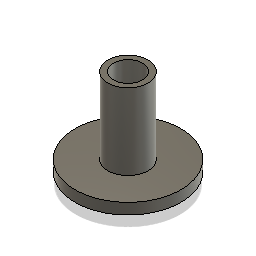
Rotor v1 (Autodesk Fusion 360 design; units mm, degrees)
Autodesk Fusion 360 part; units mm, degrees
note: some values were not read from the file. Set by a fixed rule: which sketch regions a step uses.
sketch "Esboço1" plane through (0, 0, 0) normal (0, 1, 0) x (1, 0, 0)
  circle A0 centre (0, 0) radius 14.5
  circle A1 centre (0, 0) radius 5.5
  circle A2 centre (0, 0) radius 4
  dimension "d1" = 29
  dimension "d2" = 11
  dimension "d3" = 8
  constraint coincident A0.centre A1.centre
  constraint concentric A0 A1
  measures "d1" diameter of A0
  measures "d2" diameter of A1
  measures "d3" diameter of A2
extrude "Extrusão1" add sketch "Esboço1" along normal blind 3 contours A0 makes body 1
extrude "Extrusão2" add sketch "Esboço1" against normal blind 3 separate body contours A1 makes body 2
extrude "Extrusão3" add sketch "Esboço1" along normal blind 23.8 contours A1 bodies 1 2
sketch "Esboço3" plane through (0, 0, 0) normal (0, 0, 1) x (1, 0, 0)
  line L0 (0, 0) -> (0, -7.7454)
  circle A0 centre (0, -1.6) radius 1.35
  line L1 (-1.35, -3) -> (1.35, -3)
  line L2 (-5.5, -3) -> (5.5, -3)
  line L3 (-1.35, -1.6) -> (-1.35, -3)
  line L4 (1.35, -1.6) -> (1.35, -3)
  dimension "d10" = 2.7
  dimension "d13" = 1.4
  constraint vertical L0
  constraint coincident L0 A0.centre
  constraint perpendicular L0 L1
  constraint coincident L1.start L2
  constraint coincident L0.start origin
  constraint coincident A0 L3.start
  constraint coincident A0 L4.start
  constraint parallel L3 L4
  constraint vertical L3
  constraint tangent A0 L3
  constraint tangent A0 L4
  measures "d10" diameter of A0
  measures "d13" distance of A0.centre L1
extrude "Extrusão4" cut sketch "Esboço3" along normal through all and the other way through all bodies 1
